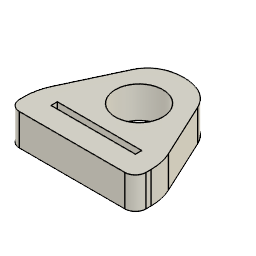
PTFE springsteel holder (Autodesk Fusion 360 design; units mm, degrees)
Autodesk Fusion 360 part; units mm, degrees
sketch "Skizze1" plane through (0, 0, 0) normal (0, 0, 1) x (1, 0, 0)
  line L0 (0, 0) -> (8, 0)
  line L1 (8, 0) -> (8, 0.6)
  line L2 (8, 0.6) -> (0, 0.6)
  line L3 (0, 0.6) -> (0, 0)
  circle A0 centre (4, 4.35) radius 2.25
  line L4 (-1, -2) -> (9, -2)
  line L5 (10, -1) -> (10, -0.5092)
  line L6 (-2, -1) -> (-2, -0.5092)
  line L7 (-1.5309, 1.6052) -> (0.8971, 6.808)
  line L8 (9.5309, 1.6052) -> (7.1029, 6.808)
  arc A1 (5.3069, 8.3939) -> (2.6931, 8.3939) centre (4, 4.3499) ccw
  arc A2 (-1.5309, 1.6052) -> (-2, -0.5092) centre (3, -0.5092) ccw
  arc A3 (10, -0.5092) -> (9.5309, 1.6052) centre (5, -0.5092) ccw
  arc A4 (-2, -1) -> (-1, -2) centre (-1, -1) ccw
  arc A5 (9, -2) -> (10, -1) centre (9, -1) ccw
  arc A6 (7.1029, 6.808) -> (5.3069, 8.3939) centre (4.3844, 5.5393) ccw
  arc A7 (2.6931, 8.3939) -> (0.8971, 6.808) centre (3.6156, 5.5393) ccw
  dimension "d1" = 8
  dimension "d2" = 0.6
  dimension "d3" = 4.5
  dimension "d14" = 5
  dimension "d15" = 5
  dimension "d16" = 1
  dimension "d17" = 1
  dimension "d18" = 3
  dimension "d19" = 3
  constraint horizontal L0
  constraint vertical L1
  constraint horizontal L2
  constraint vertical L3
  constraint coincident L0.start L3.end
  constraint tangent L6 A2
  constraint tangent L7 A2
  constraint tangent L5 A3
  constraint tangent L8 A3
  constraint tangent L4 A4
  constraint tangent L6 A4
  constraint tangent L4 A5
  constraint tangent L5 A5
  constraint tangent L8 A6
  constraint tangent A1 A6
  constraint tangent L7 A7
  constraint tangent A1 A7
  measures "d1" distance of L0.start L0.end
  measures "d2" distance of L0.start L2.end
  measures "d3" diameter of A0
  measures "d14" radius of A2
  measures "d15" radius of A3
  measures "d16" radius of A4
  measures "d17" radius of A5
  measures "d18" radius of A6
  measures "d19" radius of A7
extrude "Extrusion1" add sketch "Skizze1" along normal blind 2
extrude "Extrusion2" add 1 faces at (5.3333, -1.3333, 2) along direction (0, 0, 1) blind 1
